Autodesk Inventor part; units mm, degrees
(part 2 of 3)
  line L371 (21.6648, -2.3732) -> (20.3723, -2.3732)
  line L372 (20.3723, -2.3732) -> (20.3723, 1.7763)
  line L373 (20.3723, 1.7763) -> (21.6648, 1.7763)
  line L374 (21.6648, 1.7763) -> (21.6648, -2.3732)
  line L375 (21.7049, 2.3691) -> (20.3366, 2.3691)
  line L376 (20.3366, 2.3691) -> (20.3366, 3.3764)
  line L377 (20.3366, 3.3764) -> (21.7049, 3.3764)
  line L378 (21.7049, 3.3764) -> (21.7049, 2.3691)
  spline S238 degree 2 poles (24.9408, -1.932) (24.8071, -2.0434) (24.5976, -2.2217) (24.4193, -2.3108) knots 0 0 0 1 2 2 2
  spline S239 degree 2 poles (24.4193, -2.3108) (24.2455, -2.3955) (23.9156, -2.4847) (23.6215, -2.4847) knots 0 0 0 1 2 2 2
  spline S240 degree 2 poles (23.6215, -2.4847) (23.0688, -2.4847) (22.3423, -1.7448) (22.3423, -1.1832) knots 0 0 0 1 2 2 2
  spline S241 degree 2 poles (22.3423, -1.1832) (22.3423, -0.7241) (22.7122, -0.1536) (23.0599, 0.0113) knots 0 0 0 1 2 2 2
  spline S242 degree 2 poles (23.0599, 0.0113) (23.412, 0.1807) (24.3881, 0.3144) (24.9497, 0.35) knots 0 0 0 1 2 2 2
  line L379 (24.9497, 0.35) -> (24.9497, 0.3723)
  spline S243 degree 2 poles (24.9497, 0.3723) (24.9497, 0.7155) (24.4416, 0.9785) (23.9335, 0.9785) knots 0 0 0 1 2 2 2
  spline S244 degree 2 poles (23.9335, 0.9785) (23.7062, 0.9785) (23.0911, 0.8136) (22.8014, 0.6843) knots 0 0 0 1 2 2 2
  line L380 (22.8014, 0.6843) -> (22.69, 0.6843)
  line L381 (22.69, 0.6843) -> (22.69, 1.6871)
  spline S245 degree 2 poles (22.69, 1.6871) (22.8816, 1.7406) (23.7374, 1.8922) (24.1741, 1.8922) knots 0 0 0 1 2 2 2
  spline S246 degree 2 poles (24.1741, 1.8922) (25.2438, 1.8922) (26.2244, 1.179) (26.2244, 0.4481) knots 0 0 0 1 2 2 2
  line L382 (26.2244, 0.4481) -> (26.2244, -2.3732)
  line L383 (26.2244, -2.3732) -> (24.9408, -2.3732)
  line L384 (24.9408, -2.3732) -> (24.9408, -1.932)
  line L385 (24.9408, -1.2902) -> (24.9408, -0.43)
  spline S247 degree 2 poles (24.9408, -0.43) (24.6109, -0.4612) (24.2053, -0.5102) (24.0092, -0.5815) knots 0 0 0 1 2 2 2
  spline S248 degree 2 poles (24.0092, -0.5815) (23.8354, -0.6394) (23.6482, -0.8801) (23.6482, -1.0762) knots 0 0 0 1 2 2 2
  spline S249 degree 2 poles (23.6482, -1.0762) (23.6482, -1.3659) (23.9647, -1.5843) (24.2722, -1.5843) knots 0 0 0 1 2 2 2
  spline S250 degree 2 poles (24.2722, -1.5843) (24.4416, -1.5843) (24.7981, -1.4283) (24.9408, -1.2902) knots 0 0 0 1 2 2 2
  line L386 (31.3366, -2.3732) -> (29.7989, -2.3732)
  line L387 (29.7989, -2.3732) -> (28.6758, -0.5726)
  line L388 (28.6758, -0.5726) -> (28.4752, -0.84)
  line L389 (28.4752, -0.84) -> (28.4752, -2.3732)
  line L390 (28.4752, -2.3732) -> (27.1827, -2.3732)
  line L391 (27.1827, -2.3732) -> (27.1827, 3.3719)
  line L392 (27.1827, 3.3719) -> (28.4752, 3.3719)
  line L393 (28.4752, 3.3719) -> (28.4752, 0.1539)
  line L394 (28.4752, 0.1539) -> (29.7009, 1.7763)
  line L395 (29.7009, 1.7763) -> (31.2297, 1.7763)
  line L396 (31.2297, 1.7763) -> (29.7767, -0.011)
  line L397 (29.7767, -0.011) -> (31.3366, -2.3732)
  spline S251 degree 2 poles (-44.3619, -7.6626) (-44.3619, -8.0459) (-44.6071, -8.7412) (-44.8344, -8.973) knots 0 0 0 1 2 2 2
  spline S252 degree 2 poles (-44.8344, -8.973) (-44.9725, -9.1201) (-45.3113, -9.3608) (-45.5118, -9.4454) knots 0 0 0 1 2 2 2
  spline S253 degree 2 poles (-45.5118, -9.4454) (-45.7169, -9.5301) (-46.1938, -9.6282) (-46.4879, -9.6282) knots 0 0 0 1 2 2 2
  line L398 (-46.4879, -9.6282) -> (-47.21, -9.6282)
  line L399 (-47.21, -9.6282) -> (-47.21, -11.4288)
  line L400 (-47.21, -11.4288) -> (-48.5917, -11.4288)
  line L401 (-48.5917, -11.4288) -> (-48.5917, -5.9288)
  line L402 (-48.5917, -5.9288) -> (-46.4567, -5.9288)
  spline S254 degree 2 poles (-46.4567, -5.9288) (-45.9843, -5.9288) (-45.2934, -6.1027) (-45.0126, -6.2899) knots 0 0 0 1 2 2 2
  spline S255 degree 2 poles (-45.0126, -6.2899) (-44.7007, -6.4993) (-44.3619, -7.1857) (-44.3619, -7.6626) knots 0 0 0 1 2 2 2
  spline S256 degree 2 poles (-45.7793, -7.6983) (-45.7793, -7.4621) (-46.0021, -7.1278) (-46.1536, -7.0654) knots 0 0 0 1 2 2 2
  spline S257 degree 2 poles (-46.1536, -7.0654) (-46.3498, -6.9807) (-46.7063, -6.954) (-47.0139, -6.954) knots 0 0 0 1 2 2 2
  line L403 (-47.0139, -6.954) -> (-47.21, -6.954)
  line L404 (-47.21, -6.954) -> (-47.21, -8.6031)
  line L405 (-47.21, -8.6031) -> (-47.1119, -8.6031)
  spline S258 degree 2 poles (-47.1119, -8.6031) (-46.9203, -8.6031) (-46.5726, -8.5941) (-46.4434, -8.5719) knots 0 0 0 1 2 2 2
  spline S259 degree 2 poles (-46.4434, -8.5719) (-46.3319, -8.554) (-46.0868, -8.4471) (-46.0199, -8.3802) knots 0 0 0 1 2 2 2
  spline S260 degree 2 poles (-46.0199, -8.3802) (-45.8773, -8.2465) (-45.7793, -7.9479) (-45.7793, -7.6983) knots 0 0 0 1 2 2 2
  spline S261 degree 2 poles (-39.7177, -9.3563) (-39.7177, -10.3814) (-40.8364, -11.5581) (-41.8571, -11.5581) knots 0 0 0 1 2 2 2
  spline S262 degree 2 poles (-41.8571, -11.5581) (-42.8733, -11.5581) (-44.0009, -10.3814) (-44.0009, -9.3563) knots 0 0 0 1 2 2 2
  spline S263 degree 2 poles (-44.0009, -9.3563) (-44.0009, -8.3223) (-42.8733, -7.1501) (-41.8571, -7.1501) knots 0 0 0 1 2 2 2
  spline S264 degree 2 poles (-41.8571, -7.1501) (-40.8408, -7.1501) (-39.7177, -8.3267) (-39.7177, -9.3563) knots 0 0 0 1 2 2 2
  spline S265 degree 2 poles (-41.0414, -9.3652) (-41.0414, -8.9953) (-41.1618, -8.5006) (-41.2687, -8.3535) knots 0 0 0 1 2 2 2
  spline S266 degree 2 poles (-41.2687, -8.3535) (-41.3846, -8.1975) (-41.6743, -8.0771) (-41.8571, -8.0771) knots 0 0 0 1 2 2 2
  spline S267 degree 2 poles (-41.8571, -8.0771) (-42.0353, -8.0771) (-42.3161, -8.1841) (-42.432, -8.3356) knots 0 0 0 1 2 2 2
  spline S268 degree 2 poles (-42.432, -8.3356) (-42.5434, -8.4783) (-42.6771, -8.9819) (-42.6771, -9.3652) knots 0 0 0 1 2 2 2
  spline S269 degree 2 poles (-42.6771, -9.3652) (-42.6771, -9.7441) (-42.5524, -10.2121) (-42.4498, -10.3547) knots 0 0 0 1 2 2 2
  spline S270 degree 2 poles (-42.4498, -10.3547) (-42.3473, -10.4973) (-42.0353, -10.631) (-41.8481, -10.631) knots 0 0 0 1 2 2 2
  spline S271 degree 2 poles (-41.8481, -10.631) (-41.6921, -10.631) (-41.3712, -10.4973) (-41.2732, -10.3636) knots 0 0 0 1 2 2 2
  spline S272 degree 2 poles (-41.2732, -10.3636) (-41.1618, -10.2076) (-41.0414, -9.7574) (-41.0414, -9.3652) knots 0 0 0 1 2 2 2
  line L406 (-35.2606, -11.4288) -> (-36.5532, -11.4288)
  line L407 (-36.5532, -11.4288) -> (-36.5532, -10.9965)
  spline S273 degree 2 poles (-36.5532, -10.9965) (-36.678, -11.099) (-36.9989, -11.3352) (-37.1237, -11.3976) knots 0 0 0 1 2 2 2
  spline S274 degree 2 poles (-37.1237, -11.3976) (-37.2752, -11.4689) (-37.5783, -11.5447) (-37.7878, -11.5447) knots 0 0 0 1 2 2 2
  spline S275 degree 2 poles (-37.7878, -11.5447) (-38.4964, -11.5447) (-39.3254, -10.3681) (-39.3254, -9.3875) knots 0 0 0 1 2 2 2
  spline S276 degree 2 poles (-39.3254, -9.3875) (-39.3254, -8.8437) (-39.0447, -8.0459) (-38.7995, -7.7518) knots 0 0 0 1 2 2 2
  spline S277 degree 2 poles (-38.7995, -7.7518) (-38.5722, -7.4799) (-37.9304, -7.1679) (-37.5738, -7.1679) knots 0 0 0 1 2 2 2
  spline S278 degree 2 poles (-37.5738, -7.1679) (-37.2485, -7.1679) (-36.8295, -7.3061) (-36.5532, -7.4487) knots 0 0 0 1 2 2 2
  line L408 (-36.5532, -7.4487) -> (-36.5532, -5.6837)
  line L409 (-36.5532, -5.6837) -> (-35.2606, -5.6837)
  line L410 (-35.2606, -5.6837) -> (-35.2606, -11.4288)
  line L411 (-36.5532, -10.2878) -> (-36.5532, -8.251)
  spline S279 degree 2 poles (-36.5532, -8.251) (-36.6468, -8.2019) (-36.9588, -8.1395) (-37.0702, -8.1395) knots 0 0 0 1 2 2 2
  spline S280 degree 2 poles (-37.0702, -8.1395) (-37.5337, -8.1395) (-38.0017, -8.7903) (-38.0017, -9.3741) knots 0 0 0 1 2 2 2
  spline S281 degree 2 poles (-38.0017, -9.3741) (-38.0017, -9.9892) (-37.6273, -10.5374) (-37.2128, -10.5374) knots 0 0 0 1 2 2 2
  spline S282 degree 2 poles (-37.2128, -10.5374) (-37.0434, -10.5374) (-36.6958, -10.4037) (-36.5532, -10.2878) knots 0 0 0 1 2 2 2
  spline S283 degree 2 poles (-28.0759, -9.3563) (-28.0759, -10.3814) (-29.1946, -11.5581) (-30.2152, -11.5581) knots 0 0 0 1 2 2 2
  spline S284 degree 2 poles (-30.2152, -11.5581) (-31.2314, -11.5581) (-32.3591, -10.3814) (-32.3591, -9.3563) knots 0 0 0 1 2 2 2
  spline S285 degree 2 poles (-32.3591, -9.3563) (-32.3591, -8.3223) (-31.2314, -7.1501) (-30.2152, -7.1501) knots 0 0 0 1 2 2 2
  spline S286 degree 2 poles (-30.2152, -7.1501) (-29.199, -7.1501) (-28.0759, -8.3267) (-28.0759, -9.3563) knots 0 0 0 1 2 2 2
  spline S287 degree 2 poles (-29.3996, -9.3652) (-29.3996, -8.9953) (-29.5199, -8.5006) (-29.6269, -8.3535) knots 0 0 0 1 2 2 2
  spline S288 degree 2 poles (-29.6269, -8.3535) (-29.7428, -8.1975) (-30.0325, -8.0771) (-30.2152, -8.0771) knots 0 0 0 1 2 2 2
  spline S289 degree 2 poles (-30.2152, -8.0771) (-30.3935, -8.0771) (-30.6743, -8.1841) (-30.7902, -8.3356) knots 0 0 0 1 2 2 2
  spline S290 degree 2 poles (-30.7902, -8.3356) (-30.9016, -8.4783) (-31.0353, -8.9819) (-31.0353, -9.3652) knots 0 0 0 1 2 2 2
  spline S291 degree 2 poles (-31.0353, -9.3652) (-31.0353, -9.7441) (-30.9105, -10.2121) (-30.808, -10.3547) knots 0 0 0 1 2 2 2
  spline S292 degree 2 poles (-30.808, -10.3547) (-30.7055, -10.4973) (-30.3935, -10.631) (-30.2063, -10.631) knots 0 0 0 1 2 2 2
  spline S293 degree 2 poles (-30.2063, -10.631) (-30.0503, -10.631) (-29.7294, -10.4973) (-29.6314, -10.3636) knots 0 0 0 1 2 2 2
  spline S294 degree 2 poles (-29.6314, -10.3636) (-29.5199, -10.2076) (-29.3996, -9.7574) (-29.3996, -9.3652) knots 0 0 0 1 2 2 2
  spline S295 degree 2 poles (-23.3246, -9.2984) (-23.3246, -10.2923) (-24.3319, -11.5091) (-25.0718, -11.5091) knots 0 0 0 1 2 2 2
  spline S296 degree 2 poles (-25.0718, -11.5091) (-25.3793, -11.5091) (-25.8384, -11.3709) (-26.0969, -11.2194) knots 0 0 0 1 2 2 2
  line L412 (-26.0969, -11.2194) -> (-26.0969, -12.9487)
  line L413 (-26.0969, -12.9487) -> (-27.3895, -12.9487)
  line L414 (-27.3895, -12.9487) -> (-27.3895, -7.2793)
  line L415 (-27.3895, -7.2793) -> (-26.0969, -7.2793)
  line L416 (-26.0969, -7.2793) -> (-26.0969, -7.7161)
  spline S297 degree 2 poles (-26.0969, -7.7161) (-25.8117, -7.471) (-25.2233, -7.1679) (-24.8356, -7.1679) knots 0 0 0 1 2 2 2
  spline S298 degree 2 poles (-24.8356, -7.1679) (-24.1135, -7.1679) (-23.3246, -8.3134) (-23.3246, -9.2984) knots 0 0 0 1 2 2 2
  spline S299 degree 2 poles (-24.6484, -9.3251) (-24.6484, -8.7189) (-25.0228, -8.1752) (-25.415, -8.1752) knots 0 0 0 1 2 2 2
  spline S300 degree 2 poles (-25.415, -8.1752) (-25.5888, -8.1752) (-25.932, -8.2866) (-26.0969, -8.398) knots 0 0 0 1 2 2 2
  line L417 (-26.0969, -8.398) -> (-26.0969, -10.4795)
  spline S301 degree 2 poles (-26.0969, -10.4795) (-25.9944, -10.5241) (-25.7448, -10.5597) (-25.5754, -10.5597) knots 0 0 0 1 2 2 2
  spline S302 degree 2 poles (-25.5754, -10.5597) (-25.1075, -10.5597) (-24.6484, -9.9446) (-24.6484, -9.3251) knots 0 0 0 1 2 2 2
  line L418 (-21.3368, -11.4288) -> (-22.6293, -11.4288)
  line L419 (-22.6293, -11.4288) -> (-22.6293, -7.2793)
  line L420 (-22.6293, -7.2793) -> (-21.3368, -7.2793)
  line L421 (-21.3368, -7.2793) -> (-21.3368, -11.4288)
  line L422 (-21.2967, -6.6865) -> (-22.665, -6.6865)
  line L423 (-22.665, -6.6865) -> (-22.665, -5.6792)
  line L424 (-22.665, -5.6792) -> (-21.2967, -5.6792)
  line L425 (-21.2967, -5.6792) -> (-21.2967, -6.6865)
  spline S303 degree 2 poles (-18.2213, -11.5403) (-19.398, -11.5403) (-20.6504, -10.4171) (-20.6504, -9.3786) knots 0 0 0 1 2 2 2
  spline S304 degree 2 poles (-20.6504, -9.3786) (-20.6504, -8.3624) (-19.4827, -7.1501) (-18.4308, -7.1501) knots 0 0 0 1 2 2 2
  spline S305 degree 2 poles (-18.4308, -7.1501) (-17.4814, -7.1501) (-16.5187, -8.1796) (-16.5187, -9.1335) knots 0 0 0 1 2 2 2
  line L426 (-16.5187, -9.1335) -> (-16.5187, -9.6014)
  line L427 (-16.5187, -9.6014) -> (-19.3579, -9.6014)
  spline S306 degree 2 poles (-19.3579, -9.6014) (-19.34, -9.8911) (-19.1306, -10.2745) (-18.9612, -10.3903) knots 0 0 0 1 2 2 2
  spline S307 degree 2 poles (-18.9612, -10.3903) (-18.7963, -10.5062) (-18.3506, -10.6043) (-18.0876, -10.6043) knots 0 0 0 1 2 2 2
  spline S308 degree 2 poles (-18.0876, -10.6043) (-17.8648, -10.6043) (-17.428, -10.5062) (-17.2452, -10.4215) knots 0 0 0 1 2 2 2
  spline S309 degree 2 poles (-17.2452, -10.4215) (-17.0848, -10.3547) (-16.8173, -10.1898) (-16.7327, -10.1274) knots 0 0 0 1 2 2 2
  line L428 (-16.7327, -10.1274) -> (-16.5945, -10.1274)
  line L429 (-16.5945, -10.1274) -> (-16.5945, -11.1971)
  spline S310 degree 2 poles (-16.5945, -11.1971) (-16.7549, -11.2595) (-17.0135, -11.3664) (-17.2452, -11.4199) knots 0 0 0 1 2 2 2
  spline S311 degree 2 poles (-17.2452, -11.4199) (-17.4547, -11.4779) (-17.9004, -11.5403) (-18.2213, -11.5403) knots 0 0 0 1 2 2 2
  spline S312 degree 2 poles (-17.7934, -8.8215) (-17.8024, -8.4114) (-18.1634, -7.9791) (-18.5333, -7.9791) knots 0 0 0 1 2 2 2
  spline S313 degree 2 poles (-18.5333, -7.9791) (-18.9122, -7.9791) (-19.34, -8.4337) (-19.3623, -8.8215) knots 0 0 0 1 2 2 2
  line L430 (-19.3623, -8.8215) -> (-17.7934, -8.8215)
  line L431 (-11.7006, -11.4288) -> (-13.2383, -11.4288)
  line L432 (-13.2383, -11.4288) -> (-14.3615, -9.6282)
  line L433 (-14.3615, -9.6282) -> (-14.5621, -9.8956)
  line L434 (-14.5621, -9.8956) -> (-14.5621, -11.4288)
  line L435 (-14.5621, -11.4288) -> (-15.8546, -11.4288)
  line L436 (-15.8546, -11.4288) -> (-15.8546, -5.6837)
  line L437 (-15.8546, -5.6837) -> (-14.5621, -5.6837)
  line L438 (-14.5621, -5.6837) -> (-14.5621, -8.9017)
  line L439 (-14.5621, -8.9017) -> (-13.3364, -7.2793)
  line L440 (-13.3364, -7.2793) -> (-11.8076, -7.2793)
  line L441 (-11.8076, -7.2793) -> (-13.2606, -9.0666)
  line L442 (-13.2606, -9.0666) -> (-11.7006, -11.4288)
  spline S314 degree 2 poles (-9.0086, -10.9876) (-9.1423, -11.099) (-9.3518, -11.2773) (-9.5301, -11.3664) knots 0 0 0 1 2 2 2
  spline S315 degree 2 poles (-9.5301, -11.3664) (-9.7039, -11.4511) (-10.0337, -11.5403) (-10.3279, -11.5403) knots 0 0 0 1 2 2 2
  spline S316 degree 2 poles (-10.3279, -11.5403) (-10.8806, -11.5403) (-11.6071, -10.8004) (-11.6071, -10.2388) knots 0 0 0 1 2 2 2
  spline S317 degree 2 poles (-11.6071, -10.2388) (-11.6071, -9.7797) (-11.2371, -9.2092) (-10.8895, -9.0443) knots 0 0 0 1 2 2 2
  spline S318 degree 2 poles (-10.8895, -9.0443) (-10.5374, -8.8749) (-9.5613, -8.7412) (-8.9997, -8.7056) knots 0 0 0 1 2 2 2
  line L443 (-8.9997, -8.7056) -> (-8.9997, -8.6833)
  spline S319 degree 2 poles (-8.9997, -8.6833) (-8.9997, -8.3401) (-9.5078, -8.0771) (-10.0159, -8.0771) knots 0 0 0 1 2 2 2
  spline S320 degree 2 poles (-10.0159, -8.0771) (-10.2432, -8.0771) (-10.8583, -8.242) (-11.148, -8.3713) knots 0 0 0 1 2 2 2
  line L444 (-11.148, -8.3713) -> (-11.2594, -8.3713)
  line L445 (-11.2594, -8.3713) -> (-11.2594, -7.3685)
  spline S321 degree 2 poles (-11.2594, -7.3685) (-11.0677, -7.315) (-10.212, -7.1634) (-9.7752, -7.1634) knots 0 0 0 1 2 2 2
  spline S322 degree 2 poles (-9.7752, -7.1634) (-8.7055, -7.1634) (-7.725, -7.8766) (-7.725, -8.6075) knots 0 0 0 1 2 2 2
  line L446 (-7.725, -8.6075) -> (-7.725, -11.4288)
  line L447 (-7.725, -11.4288) -> (-9.0086, -11.4288)
  line L448 (-9.0086, -11.4288) -> (-9.0086, -10.9876)
  spline S323 degree 2 poles (-7.9746, -11.4288) (-8.1127, -11.5358) (-8.2464, -11.7676) (-8.2464, -11.8745) knots 0 0 0 1 2 2 2
  spline S324 degree 2 poles (-8.2464, -11.8745) (-8.2464, -11.9191) (-8.2197, -11.9993) (-8.1885, -12.035) knots 0 0 0 1 2 2 2
  spline S325 degree 2 poles (-8.1885, -12.035) (-8.1484, -12.0751) (-8.0637, -12.1152) (-7.9835, -12.1152) knots 0 0 0 1 2 2 2
  spline S326 degree 2 poles (-7.9835, -12.1152) (-7.93, -12.1152) (-7.8007, -12.084) (-7.7562, -12.0706) knots 0 0 0 1 2 2 2
  line L449 (-7.7562, -12.0706) -> (-7.7205, -12.0706)
  line L450 (-7.7205, -12.0706) -> (-7.7205, -12.8373)
  spline S327 degree 2 poles (-7.7205, -12.8373) (-7.872, -12.8952) (-8.2687, -12.9487) (-8.3846, -12.9487) knots 0 0 0 1 2 2 2
  spline S328 degree 2 poles (-8.3846, -12.9487) (-8.7323, -12.9487) (-9.1646, -12.5832) (-9.1646, -12.3113) knots 0 0 0 1 2 2 2
  spline S329 degree 2 poles (-9.1646, -12.3113) (-9.1646, -12.0305) (-8.8972, -11.567) (-8.7367, -11.4288) knots 0 0 0 1 2 2 2
  line L451 (-8.7367, -11.4288) -> (-7.9746, -11.4288)
  line L452 (-9.0086, -10.3458) -> (-9.0086, -9.4856)
  spline S330 degree 2 poles (-9.0086, -9.4856) (-9.3384, -9.5168) (-9.744, -9.5658) (-9.9401, -9.6371) knots 0 0 0 1 2 2 2
  spline S331 degree 2 poles (-9.9401, -9.6371) (-10.1139, -9.695) (-10.3011, -9.9357) (-10.3011, -10.1318) knots 0 0 0 1 2 2 2
  spline S332 degree 2 poles (-10.3011, -10.1318) (-10.3011, -10.4215) (-9.9847, -10.6399) (-9.6771, -10.6399) knots 0 0 0 1 2 2 2
  spline S333 degree 2 poles (-9.6771, -10.6399) (-9.5078, -10.6399) (-9.1512, -10.4839) (-9.0086, -10.3458) knots 0 0 0 1 2 2 2
  line L453 (0.4002, -11.4288) -> (0.4002, -9.3563)
  spline S334 degree 2 poles (0.4002, -9.3563) (0.4002, -9.0488) (0.378, -8.6298) (0.3245, -8.4961) knots 0 0 0 1 2 2 2
  spline S335 degree 2 poles (0.3245, -8.4961) (0.2665, -8.3624) (0.0348, -8.242) (-0.1747, -8.242) knots 0 0 0 1 2 2 2
  spline S336 degree 2 poles (-0.1747, -8.242) (-0.3218, -8.242) (-0.6071, -8.3713) (-0.7764, -8.4916) knots 0 0 0 1 2 2 2
  line L454 (-0.7764, -8.4916) -> (-0.7764, -11.4288)
  line L455 (-0.7764, -11.4288) -> (-2.0779, -11.4288)
  line L456 (-2.0779, -11.4288) -> (-2.0779, -9.3563)
  spline S337 degree 2 poles (-2.0779, -9.3563) (-2.0779, -9.0532) (-2.1046, -8.6298) (-2.1581, -8.4961) knots 0 0 0 1 2 2 2
  spline S338 degree 2 poles (-2.1581, -8.4961) (-2.216, -8.3624) (-2.4478, -8.242) (-2.6573, -8.242) knots 0 0 0 1 2 2 2
  spline S339 degree 2 poles (-2.6573, -8.242) (-2.8133, -8.242) (-3.1208, -8.3891) (-3.2635, -8.4916) knots 0 0 0 1 2 2 2
  line L457 (-3.2635, -8.4916) -> (-3.2635, -11.4288)
  line L458 (-3.2635, -11.4288) -> (-4.556, -11.4288)
  line L459 (-4.556, -11.4288) -> (-4.556, -7.2793)
  line L460 (-4.556, -7.2793) -> (-3.2635, -7.2793)
  line L461 (-3.2635, -7.2793) -> (-3.2635, -7.7384)
  spline S340 degree 2 poles (-3.2635, -7.7384) (-2.947, -7.471) (-2.381, -7.1679) (-2.0289, -7.1679) knots 0 0 0 1 2 2 2
  spline S341 degree 2 poles (-2.0289, -7.1679) (-1.65, -7.1679) (-1.0706, -7.5289) (-0.919, -7.8899) knots 0 0 0 1 2 2 2
  spline S342 degree 2 poles (-0.919, -7.8899) (-0.5491, -7.5423) (0.1105, -7.1679) (0.4493, -7.1679) knots 0 0 0 1 2 2 2
  spline S343 degree 2 poles (0.4493, -7.1679) (0.739, -7.1679) (1.1981, -7.3506) (1.3541, -7.5378) knots 0 0 0 1 2 2 2
  spline S344 degree 2 poles (1.3541, -7.5378) (1.5279, -7.7384) (1.7017, -8.2866) (1.7017, -8.7279) knots 0 0 0 1 2 2 2
  line L462 (1.7017, -8.7279) -> (1.7017, -11.4288)
  line L463 (1.7017, -11.4288) -> (0.4002, -11.4288)
  spline S345 degree 2 poles (4.786, -11.5403) (3.6093, -11.5403) (2.3569, -10.4171) (2.3569, -9.3786) knots 0 0 0 1 2 2 2
  spline S346 degree 2 poles (2.3569, -9.3786) (2.3569, -8.3624) (3.5246, -7.1501) (4.5765, -7.1501) knots 0 0 0 1 2 2 2
  spline S347 degree 2 poles (4.5765, -7.1501) (5.5259, -7.1501) (6.4886, -8.1796) (6.4886, -9.1335) knots 0 0 0 1 2 2 2
  line L464 (6.4886, -9.1335) -> (6.4886, -9.6014)
  line L465 (6.4886, -9.6014) -> (3.6494, -9.6014)
  spline S348 degree 2 poles (3.6494, -9.6014) (3.6673, -9.8911) (3.8767, -10.2745) (4.0461, -10.3903) knots 0 0 0 1 2 2 2
  spline S349 degree 2 poles (4.0461, -10.3903) (4.211, -10.5062) (4.6567, -10.6043) (4.9197, -10.6043) knots 0 0 0 1 2 2 2
  spline S350 degree 2 poles (4.9197, -10.6043) (5.1425, -10.6043) (5.5793, -10.5062) (5.7621, -10.4215) knots 0 0 0 1 2 2 2
  spline S351 degree 2 poles (5.7621, -10.4215) (5.9225, -10.3547) (6.19, -10.1898) (6.2746, -10.1274) knots 0 0 0 1 2 2 2
  line L466 (6.2746, -10.1274) -> (6.4128, -10.1274)
  line L467 (6.4128, -10.1274) -> (6.4128, -11.1971)
  spline S352 degree 2 poles (6.4128, -11.1971) (6.2523, -11.2595) (5.9938, -11.3664) (5.7621, -11.4199) knots 0 0 0 1 2 2 2
  spline S353 degree 2 poles (5.7621, -11.4199) (5.5526, -11.4779) (5.1069, -11.5403) (4.786, -11.5403) knots 0 0 0 1 2 2 2
  spline S354 degree 2 poles (5.2139, -8.8215) (5.2049, -8.4114) (4.8439, -7.9791) (4.474, -7.9791) knots 0 0 0 1 2 2 2
  spline S355 degree 2 poles (4.474, -7.9791) (4.0951, -7.9791) (3.6673, -8.4337) (3.645, -8.8215) knots 0 0 0 1 2 2 2
  line L468 (3.645, -8.8215) -> (5.2139, -8.8215)
  line L469 (9.9383, -8.505) -> (9.8314, -8.505)
  spline S356 degree 2 poles (9.8314, -8.505) (9.7556, -8.4783) (9.4748, -8.4515) (9.3054, -8.4515) knots 0 0 0 1 2 2 2
  spline S357 degree 2 poles (9.3054, -8.4515) (9.1049, -8.4515) (8.6547, -8.5719) (8.4452, -8.6521) knots 0 0 0 1 2 2 2
  line L470 (8.4452, -8.6521) -> (8.4452, -11.4288)
  line L471 (8.4452, -11.4288) -> (7.1527, -11.4288)
  line L472 (7.1527, -11.4288) -> (7.1527, -7.2793)
  line L473 (7.1527, -7.2793) -> (8.4452, -7.2793)
  line L474 (8.4452, -7.2793) -> (8.4452, -7.8766)
  spline S358 degree 2 poles (8.4452, -7.8766) (8.5344, -7.7963) (8.8464, -7.5467) (8.9756, -7.471) knots 0 0 0 1 2 2 2
  spline S359 degree 2 poles (8.9756, -7.471) (9.1182, -7.3863) (9.4926, -7.2659) (9.6575, -7.2659) knots 0 0 0 1 2 2 2
  spline S360 degree 2 poles (9.6575, -7.2659) (9.7199, -7.2659) (9.8759, -7.2749) (9.9383, -7.2793) knots 0 0 0 1 2 2 2
  line L475 (9.9383, -7.2793) -> (9.9383, -8.505)
  line L476 (14.3018, -7.2793) -> (12.2114, -12.9487)
  line L477 (12.2114, -12.9487) -> (10.8208, -12.9487)
  line L478 (10.8208, -12.9487) -> (11.4493, -11.3263)
  line L479 (11.4493, -11.3263) -> (9.9294, -7.2793)
  line L480 (9.9294, -7.2793) -> (11.2844, -7.2793)
  line L481 (11.2844, -7.2793) -> (12.1579, -9.8822)
  line L482 (12.1579, -9.8822) -> (12.9736, -7.2793)
  line L483 (12.9736, -7.2793) -> (14.3018, -7.2793)
  spline S361 degree 2 poles (16.3743, -11.5091) (15.5854, -11.5091) (14.8634, -10.8583) (14.8634, -10.1185) knots 0 0 0 1 2 2 2
  line L484 (14.8634, -10.1185) -> (14.8634, -8.1796)
  line L485 (14.8634, -8.1796) -> (14.3686, -8.1796)
  line L486 (14.3686, -8.1796) -> (14.3686, -7.2793)
  line L487 (14.3686, -7.2793) -> (14.8634, -7.2793)
  line L488 (14.8634, -7.2793) -> (14.8634, -6.0937)
  line L489 (14.8634, -6.0937) -> (16.1559, -6.0937)
  line L490 (16.1559, -6.0937) -> (16.1559, -7.2793)
  line L491 (16.1559, -7.2793) -> (17.4039, -7.2793)
  line L492 (17.4039, -7.2793) -> (17.4039, -8.1796)
  line L493 (17.4039, -8.1796) -> (16.1559, -8.1796)
  line L494 (16.1559, -8.1796) -> (16.1559, -9.6549)
  spline S362 degree 2 poles (16.1559, -9.6549) (16.1559, -9.8733) (16.1648, -10.1987) (16.2183, -10.3279) knots 0 0 0 1 2 2 2
  spline S363 degree 2 poles (16.2183, -10.3279) (16.2718, -10.4572) (16.5348, -10.6087) (16.7844, -10.6087) knots 0 0 0 1 2 2 2
  spline S364 degree 2 poles (16.7844, -10.6087) (16.8913, -10.6087) (17.2256, -10.5196) (17.2925, -10.4839) knots 0 0 0 1 2 2 2
  line L495 (17.2925, -10.4839) -> (17.4039, -10.4839)
  line L496 (17.4039, -10.4839) -> (17.4039, -11.3932)
  spline S365 degree 2 poles (17.4039, -11.3932) (17.1944, -11.4467) (16.722, -11.5091) (16.3743, -11.5091) knots 0 0 0 1 2 2 2
  spline S366 degree 2 poles (21.91, -9.3563) (21.91, -10.3814) (20.7912, -11.5581) (19.7706, -11.5581) knots 0 0 0 1 2 2 2
  spline S367 degree 2 poles (19.7706, -11.5581) (18.7544, -11.5581) (17.6267, -10.3814) (17.6267, -9.3563) knots 0 0 0 1 2 2 2
  spline S368 degree 2 poles (17.6267, -9.3563) (17.6267, -8.3223) (18.7544, -7.1501) (19.7706, -7.1501) knots 0 0 0 1 2 2 2
  spline S369 degree 2 poles (19.7706, -7.1501) (20.7868, -7.1501) (21.91, -8.3267) (21.91, -9.3563) knots 0 0 0 1 2 2 2
  spline S370 degree 2 poles (20.5862, -9.3652) (20.5862, -8.9953) (20.4659, -8.5006) (20.3589, -8.3535) knots 0 0 0 1 2 2 2
  spline S371 degree 2 poles (20.3589, -8.3535) (20.243, -8.1975) (19.9533, -8.0771) (19.7706, -8.0771) knots 0 0 0 1 2 2 2
  spline S372 degree 2 poles (19.7706, -8.0771) (19.5923, -8.0771) (19.3115, -8.1841) (19.1956, -8.3356) knots 0 0 0 1 2 2 2
  spline S373 degree 2 poles (19.1956, -8.3356) (19.0842, -8.4783) (18.9505, -8.9819) (18.9505, -9.3652) knots 0 0 0 1 2 2 2
  spline S374 degree 2 poles (18.9505, -9.3652) (18.9505, -9.7441) (19.0753, -10.2121) (19.1778, -10.3547) knots 0 0 0 1 2 2 2
  spline S375 degree 2 poles (19.1778, -10.3547) (19.2803, -10.4973) (19.5923, -10.631) (19.7795, -10.631) knots 0 0 0 1 2 2 2
  spline S376 degree 2 poles (19.7795, -10.631) (19.9355, -10.631) (20.2564, -10.4973) (20.3545, -10.3636) knots 0 0 0 1 2 2 2
  spline S377 degree 2 poles (20.3545, -10.3636) (20.4659, -10.2076) (20.5862, -9.7574) (20.5862, -9.3652) knots 0 0 0 1 2 2 2
  line L497 (25.382, -8.505) -> (25.275, -8.505)
  spline S378 degree 2 poles (25.275, -8.505) (25.1993, -8.4783) (24.9185, -8.4515) (24.7491, -8.4515) knots 0 0 0 1 2 2 2
  spline S379 degree 2 poles (24.7491, -8.4515) (24.5485, -8.4515) (24.0984, -8.5719) (23.8889, -8.6521) knots 0 0 0 1 2 2 2
  line L498 (23.8889, -8.6521) -> (23.8889, -11.4288)
  line L499 (23.8889, -11.4288) -> (22.5964, -11.4288)
  line L500 (22.5964, -11.4288) -> (22.5964, -7.2793)
  line L501 (22.5964, -7.2793) -> (23.8889, -7.2793)
  line L502 (23.8889, -7.2793) -> (23.8889, -7.8766)
  spline S380 degree 2 poles (23.8889, -7.8766) (23.978, -7.7963) (24.29, -7.5467) (24.4193, -7.471) knots 0 0 0 1 2 2 2
  spline S381 degree 2 poles (24.4193, -7.471) (24.5619, -7.3863) (24.9363, -7.2659) (25.1012, -7.2659) knots 0 0 0 1 2 2 2
  spline S382 degree 2 poles (25.1012, -7.2659) (25.1636, -7.2659) (25.3196, -7.2749) (25.382, -7.2793) knots 0 0 0 1 2 2 2
  line L503 (25.382, -7.2793) -> (25.382, -8.505)
  line L504 (29.7455, -7.2793) -> (27.6551, -12.9487)
  line L505 (27.6551, -12.9487) -> (26.2645, -12.9487)
  line L506 (26.2645, -12.9487) -> (26.8929, -11.3263)
  line L507 (26.8929, -11.3263) -> (25.3731, -7.2793)
  line L508 (25.3731, -7.2793) -> (26.728, -7.2793)
  line L509 (26.728, -7.2793) -> (27.6016, -9.8822)
  line L510 (27.6016, -9.8822) -> (28.4173, -7.2793)
  line L511 (28.4173, -7.2793) -> (29.7455, -7.2793)
  spline S383 degree 2 poles (32.2637, -11.5403) (31.7511, -11.5403) (30.8998, -11.2817) (30.5834, -11.0143) knots 0 0 0 1 2 2 2
  spline S384 degree 2 poles (30.5834, -11.0143) (30.2759, -10.7424) (29.9282, -9.9268) (29.9282, -9.3741) knots 0 0 0 1 2 2 2
  spline S385 degree 2 poles (29.9282, -9.3741) (29.9282, -8.7769) (30.3026, -7.9434) (30.628, -7.676) knots 0 0 0 1 2 2 2
  spline S386 degree 2 poles (30.628, -7.676) (30.9355, -7.4175) (31.7734, -7.1679) (32.228, -7.1679) knots 0 0 0 1 2 2 2
  spline S387 degree 2 poles (32.228, -7.1679) (32.5712, -7.1679) (33.2576, -7.3283) (33.6053, -7.5022) knots 0 0 0 1 2 2 2
  line L512 (33.6053, -7.5022) -> (33.6053, -8.6075)
  line L513 (33.6053, -8.6075) -> (33.4404, -8.6075)
  spline S388 degree 2 poles (33.4404, -8.6075) (33.3601, -8.5317) (33.1373, -8.3535) (33.0036, -8.2822) knots 0 0 0 1 2 2 2
  spline S389 degree 2 poles (33.0036, -8.2822) (32.8609, -8.2019) (32.5088, -8.095) (32.2904, -8.095) knots 0 0 0 1 2 2 2
  spline S390 degree 2 poles (32.2904, -8.095) (31.7957, -8.095) (31.2519, -8.7858) (31.2519, -9.3741) knots 0 0 0 1 2 2 2
  spline S391 degree 2 poles (31.2519, -9.3741) (31.2519, -9.9981) (31.8314, -10.6132) (32.3127, -10.6132) knots 0 0 0 1 2 2 2
  spline S392 degree 2 poles (32.3127, -10.6132) (32.5579, -10.6132) (32.9233, -10.5018) (33.0571, -10.4215) knots 0 0 0 1 2 2 2
  spline S393 degree 2 poles (33.0571, -10.4215) (33.1863, -10.3458) (33.3735, -10.1764) (33.4404, -10.1095) knots 0 0 0 1 2 2 2
  line L514 (33.4404, -10.1095) -> (33.6053, -10.1095)
  line L515 (33.6053, -10.1095) -> (33.6053, -11.2194)
  spline S394 degree 2 poles (33.6053, -11.2194) (33.4938, -11.2684) (33.2041, -11.3932) (33.0526, -11.4333) knots 0 0 0 1 2 2 2
  spline S395 degree 2 poles (33.0526, -11.4333) (32.8654, -11.4868) (32.5356, -11.5403) (32.2637, -11.5403) knots 0 0 0 1 2 2 2
  line L516 (37.5275, -11.4288) -> (33.9039, -11.4288)
  line L517 (33.9039, -11.4288) -> (33.9039, -10.5775)
  line L518 (33.9039, -10.5775) -> (35.8828, -8.251)
  line L519 (35.8828, -8.251) -> (33.993, -8.251)
  line L520 (33.993, -8.251) -> (33.993, -7.2793)
  line L521 (33.993, -7.2793) -> (37.4874, -7.2793)
  line L522 (37.4874, -7.2793) -> (37.4874, -8.1172)
  line L523 (37.4874, -8.1172) -> (35.504, -10.4394)
  line L524 (35.504, -10.4394) -> (37.5275, -10.4394)
  line L525 (37.5275, -10.4394) -> (37.5275, -11.4288)
  line L526 (42.0781, -11.4288) -> (40.7767, -11.4288)
  line L527 (40.7767, -11.4288) -> (40.7767, -9.3741)
  spline S396 degree 2 poles (40.7767, -9.3741) (40.7767, -9.1201) (40.7365, -8.6209) (40.6831, -8.505) knots 0 0 0 1 2 2 2
  spline S397 degree 2 poles (40.6831, -8.505) (40.6162, -8.3624) (40.3666, -8.242) (40.1527, -8.242) knots 0 0 0 1 2 2 2
  spline S398 degree 2 poles (40.1527, -8.242) (39.9967, -8.242) (39.6713, -8.3624) (39.4886, -8.4916) knots 0 0 0 1 2 2 2
  line L528 (39.4886, -8.4916) -> (39.4886, -11.4288)
  line L529 (39.4886, -11.4288) -> (38.196, -11.4288)
  line L530 (38.196, -11.4288) -> (38.196, -7.2793)
  line L531 (38.196, -7.2793) -> (39.4886, -7.2793)
  line L532 (39.4886, -7.2793) -> (39.4886, -7.7384)
  spline S399 degree 2 poles (39.4886, -7.7384) (39.805, -7.471) (40.4067, -7.1679) (40.7722, -7.1679) knots 0 0 0 1 2 2 2
  spline S400 degree 2 poles (40.7722, -7.1679) (41.4051, -7.1679) (42.0781, -7.9702) (42.0781, -8.7279) knots 0 0 0 1 2 2 2
  line L533 (42.0781, -8.7279) -> (42.0781, -11.4288)
  spline S401 degree 2 poles (45.3229, -10.9876) (45.1891, -11.099) (44.9797, -11.2773) (44.8014, -11.3664) knots 0 0 0 1 2 2 2
  spline S402 degree 2 poles (44.8014, -11.3664) (44.6276, -11.4511) (44.2977, -11.5403) (44.0036, -11.5403) knots 0 0 0 1 2 2 2
  spline S403 degree 2 poles (44.0036, -11.5403) (43.4509, -11.5403) (42.7244, -10.8004) (42.7244, -10.2388) knots 0 0 0 1 2 2 2
  spline S404 degree 2 poles (42.7244, -10.2388) (42.7244, -9.7797) (43.0943, -9.2092) (43.442, -9.0443) knots 0 0 0 1 2 2 2
  spline S405 degree 2 poles (43.442, -9.0443) (43.7941, -8.8749) (44.7702, -8.7412) (45.3318, -8.7056) knots 0 0 0 1 2 2 2
  line L534 (45.3318, -8.7056) -> (45.3318, -8.6833)
  spline S406 degree 2 poles (45.3318, -8.6833) (45.3318, -8.3401) (44.8237, -8.0771) (44.3156, -8.0771) knots 0 0 0 1 2 2 2
  spline S407 degree 2 poles (44.3156, -8.0771) (44.0882, -8.0771) (43.4732, -8.242) (43.1835, -8.3713) knots 0 0 0 1 2 2 2
  line L535 (43.1835, -8.3713) -> (43.072, -8.3713)
  line L536 (43.072, -8.3713) -> (43.072, -7.3685)
  spline S408 degree 2 poles (43.072, -7.3685) (43.2637, -7.315) (44.1194, -7.1634) (44.5562, -7.1634) knots 0 0 0 1 2 2 2
  spline S409 degree 2 poles (44.5562, -7.1634) (45.6259, -7.1634) (46.6065, -7.8766) (46.6065, -8.6075) knots 0 0 0 1 2 2 2
  line L537 (46.6065, -8.6075) -> (46.6065, -11.4288)
  line L538 (46.6065, -11.4288) -> (45.3229, -11.4288)
  line L539 (45.3229, -11.4288) -> (45.3229, -10.9876)
  spline S410 degree 2 poles (46.3569, -11.4288) (46.2187, -11.5358) (46.085, -11.7676) (46.085, -11.8745) knots 0 0 0 1 2 2 2
  spline S411 degree 2 poles (46.085, -11.8745) (46.085, -11.9191) (46.1118, -11.9993) (46.1429, -12.035) knots 0 0 0 1 2 2 2
  spline S412 degree 2 poles (46.1429, -12.035) (46.1831, -12.0751) (46.2677, -12.1152) (46.348, -12.1152) knots 0 0 0 1 2 2 2
  spline S413 degree 2 poles (46.348, -12.1152) (46.4015, -12.1152) (46.5307, -12.084) (46.5753, -12.0706) knots 0 0 0 1 2 2 2
  line L540 (46.5753, -12.0706) -> (46.6109, -12.0706)
  line L541 (46.6109, -12.0706) -> (46.6109, -12.8373)
  spline S414 degree 2 poles (46.6109, -12.8373) (46.4594, -12.8952) (46.0627, -12.9487) (45.9468, -12.9487) knots 0 0 0 1 2 2 2
  spline S415 degree 2 poles (45.9468, -12.9487) (45.5992, -12.9487) (45.1669, -12.5832) (45.1669, -12.3113) knots 0 0 0 1 2 2 2
  spline S416 degree 2 poles (45.1669, -12.3113) (45.1669, -12.0305) (45.4343, -11.567) (45.5947, -11.4288) knots 0 0 0 1 2 2 2
  line L542 (45.5947, -11.4288) -> (46.3569, -11.4288)
  line L543 (45.3229, -10.3458) -> (45.3229, -9.4856)
  spline S417 degree 2 poles (45.3229, -9.4856) (44.993, -9.5168) (44.5874, -9.5658) (44.3913, -9.6371) knots 0 0 0 1 2 2 2
  spline S418 degree 2 poles (44.3913, -9.6371) (44.2175, -9.695) (44.0303, -9.9357) (44.0303, -10.1318) knots 0 0 0 1 2 2 2
  spline S419 degree 2 poles (44.0303, -10.1318) (44.0303, -10.4215) (44.3468, -10.6399) (44.6543, -10.6399) knots 0 0 0 1 2 2 2
  spline S420 degree 2 poles (44.6543, -10.6399) (44.8237, -10.6399) (45.1802, -10.4839) (45.3229, -10.3458) knots 0 0 0 1 2 2 2
  line L544 (49.098, -8.7323) -> (47.7921, -8.7323)
  line L545 (47.7921, -8.7323) -> (47.7921, -7.2793)
  line L546 (47.7921, -7.2793) -> (49.098, -7.2793)
  line L547 (49.098, -7.2793) -> (49.098, -8.7323)
  line L548 (49.098, -11.4288) -> (47.7921, -11.4288)
  line L549 (47.7921, -11.4288) -> (47.7921, -9.9758)
  line L550 (47.7921, -9.9758) -> (49.098, -9.9758)
  line L551 (49.098, -9.9758) -> (49.098, -11.4288)
  line L552 (-53.2604, -20.4844) -> (-54.553, -20.4844)
  line L553 (-54.553, -20.4844) -> (-54.553, -20.0521)
  spline S421 degree 2 poles (-54.553, -20.0521) (-54.6778, -20.1546) (-54.9987, -20.3908) (-55.1235, -20.4532) knots 0 0 0 1 2 2 2
  spline S422 degree 2 poles (-55.1235, -20.4532) (-55.275, -20.5246) (-55.5781, -20.6003) (-55.7876, -20.6003) knots 0 0 0 1 2 2 2
  spline S423 degree 2 poles (-55.7876, -20.6003) (-56.4962, -20.6003) (-57.3252, -19.4237) (-57.3252, -18.4431) knots 0 0 0 1 2 2 2
  spline S424 degree 2 poles (-57.3252, -18.4431) (-57.3252, -17.8993) (-57.0444, -17.1015) (-56.7993, -16.8074) knots 0 0 0 1 2 2 2
  spline S425 degree 2 poles (-56.7993, -16.8074) (-56.572, -16.5355) (-55.9302, -16.2235) (-55.5736, -16.2235) knots 0 0 0 1 2 2 2
  spline S426 degree 2 poles (-55.5736, -16.2235) (-55.2483, -16.2235) (-54.8293, -16.3617) (-54.553, -16.5043) knots 0 0 0 1 2 2 2
  line L554 (-54.553, -16.5043) -> (-54.553, -14.7393)
  line L555 (-54.553, -14.7393) -> (-53.2604, -14.7393)
  line L556 (-53.2604, -14.7393) -> (-53.2604, -20.4844)
  line L557 (-54.553, -19.3434) -> (-54.553, -17.3066)
  spline S427 degree 2 poles (-54.553, -17.3066) (-54.6466, -17.2575) (-54.9585, -17.1951) (-55.07, -17.1951) knots 0 0 0 1 2 2 2
  spline S428 degree 2 poles (-55.07, -17.1951) (-55.5335, -17.1951) (-56.0015, -17.8459) (-56.0015, -18.4297) knots 0 0 0 1 2 2 2
  spline S429 degree 2 poles (-56.0015, -18.4297) (-56.0015, -19.0448) (-55.6271, -19.593) (-55.2126, -19.593) knots 0 0 0 1 2 2 2
  spline S430 degree 2 poles (-55.2126, -19.593) (-55.0432, -19.593) (-54.6956, -19.4593) (-54.553, -19.3434) knots 0 0 0 1 2 2 2
  line L558 (-49.4853, -17.5606) -> (-49.5923, -17.5606)
  spline S431 degree 2 poles (-49.5923, -17.5606) (-49.668, -17.5339) (-49.9488, -17.5071) (-50.1182, -17.5071) knots 0 0 0 1 2 2 2
  spline S432 degree 2 poles (-50.1182, -17.5071) (-50.3188, -17.5071) (-50.7689, -17.6275) (-50.9784, -17.7077) knots 0 0 0 1 2 2 2
  line L559 (-50.9784, -17.7077) -> (-50.9784, -20.4844)
  line L560 (-50.9784, -20.4844) -> (-52.2709, -20.4844)
  line L561 (-52.2709, -20.4844) -> (-52.2709, -16.3349)
  line L562 (-52.2709, -16.3349) -> (-50.9784, -16.3349)
  line L563 (-50.9784, -16.3349) -> (-50.9784, -16.9322)
  spline S433 degree 2 poles (-50.9784, -16.9322) (-50.8893, -16.8519) (-50.5773, -16.6023) (-50.448, -16.5266) knots 0 0 0 1 2 2 2
  spline S434 degree 2 poles (-50.448, -16.5266) (-50.3054, -16.4419) (-49.931, -16.3216) (-49.7661, -16.3216) knots 0 0 0 1 2 2 2
  spline S435 degree 2 poles (-49.7661, -16.3216) (-49.7037, -16.3216) (-49.5477, -16.3305) (-49.4853, -16.3349) knots 0 0 0 1 2 2 2
  line L564 (-49.4853, -16.3349) -> (-49.4853, -17.5606)
  line L565 (-45.4829, -20.4844) -> (-46.7754, -20.4844)
  line L566 (-46.7754, -20.4844) -> (-46.7754, -16.3349)
  line L567 (-46.7754, -16.3349) -> (-45.4829, -16.3349)
  line L568 (-45.4829, -16.3349) -> (-45.4829, -20.4844)
  line L569 (-45.4427, -15.7421) -> (-46.8111, -15.7421)
  line L570 (-46.8111, -15.7421) -> (-46.8111, -14.7348)
  line L571 (-46.8111, -14.7348) -> (-45.4427, -14.7348)
  line L572 (-45.4427, -14.7348) -> (-45.4427, -15.7421)
  line L573 (-40.6113, -20.4844) -> (-41.9128, -20.4844)
  line L574 (-41.9128, -20.4844) -> (-41.9128, -18.4297)
  spline S436 degree 2 poles (-41.9128, -18.4297) (-41.9128, -18.1757) (-41.9529, -17.6765) (-42.0064, -17.5606) knots 0 0 0 1 2 2 2
  spline S437 degree 2 poles (-42.0064, -17.5606) (-42.0732, -17.418) (-42.3228, -17.2976) (-42.5367, -17.2976) knots 0 0 0 1 2 2 2
  spline S438 degree 2 poles (-42.5367, -17.2976) (-42.6927, -17.2976) (-43.0181, -17.418) (-43.2009, -17.5472) knots 0 0 0 1 2 2 2
  line L575 (-43.2009, -17.5472) -> (-43.2009, -20.4844)
  line L576 (-43.2009, -20.4844) -> (-44.4934, -20.4844)
  line L577 (-44.4934, -20.4844) -> (-44.4934, -16.3349)
  line L578 (-44.4934, -16.3349) -> (-43.2009, -16.3349)
  line L579 (-43.2009, -16.3349) -> (-43.2009, -16.794)
  spline S439 degree 2 poles (-43.2009, -16.794) (-42.8844, -16.5266) (-42.2827, -16.2235) (-41.9172, -16.2235) knots 0 0 0 1 2 2 2
  spline S440 degree 2 poles (-41.9172, -16.2235) (-41.2843, -16.2235) (-40.6113, -17.0258) (-40.6113, -17.7835) knots 0 0 0 1 2 2 2
  line L580 (-40.6113, -17.7835) -> (-40.6113, -20.4844)
  line L581 (-36.3459, -20.4844) -> (-39.9695, -20.4844)
  line L582 (-39.9695, -20.4844) -> (-39.9695, -19.6331)
  line L583 (-39.9695, -19.6331) -> (-37.9906, -17.3066)
  line L584 (-37.9906, -17.3066) -> (-39.8803, -17.3066)
  line L585 (-39.8803, -17.3066) -> (-39.8803, -16.3349)
  line L586 (-39.8803, -16.3349) -> (-36.386, -16.3349)
  line L587 (-36.386, -16.3349) -> (-36.386, -17.1728)
  line L588 (-36.386, -17.1728) -> (-38.3694, -19.495)
  line L589 (-38.3694, -19.495) -> (-36.3459, -19.495)
  line L590 (-36.3459, -19.495) -> (-36.3459, -20.4844)
  line L591 (-37.4245, -15.7466) -> (-38.7527, -15.7466)
  line L592 (-38.7527, -15.7466) -> (-38.7527, -14.7393)
  line L593 (-38.7527, -14.7393) -> (-37.4245, -14.7393)
  line L594 (-37.4245, -14.7393) -> (-37.4245, -15.7466)
  line L595 (-34.3402, -20.4844) -> (-35.6461, -20.4844)
  line L596 (-35.6461, -20.4844) -> (-35.6461, -19.0314)
  line L597 (-35.6461, -19.0314) -> (-34.3402, -19.0314)
  line L598 (-34.3402, -19.0314) -> (-34.3402, -20.4844)
  spline S441 degree 2 poles (-26.117, -17.7389) (-26.117, -18.51) (-26.79, -19.7223) (-27.3026, -20.0476) knots 0 0 0 1 2 2 2
  spline S442 degree 2 poles (-27.3026, -20.0476) (-27.7304, -20.324) (-28.7377, -20.4844) (-29.3038, -20.4844) knots 0 0 0 1 2 2 2
  line L599 (-29.3038, -20.4844) -> (-31.0242, -20.4844)
  line L600 (-31.0242, -20.4844) -> (-31.0242, -14.9844)
  line L601 (-31.0242, -14.9844) -> (-29.3216, -14.9844)
  spline S443 degree 2 poles (-29.3216, -14.9844) (-28.7422, -14.9844) (-27.7304, -15.1315) (-27.2847, -15.4168) knots 0 0 0 1 2 2 2
  spline S444 degree 2 poles (-27.2847, -15.4168) (-26.7454, -15.7644) (-26.117, -16.9411) (-26.117, -17.7389) knots 0 0 0 1 2 2 2
  spline S445 degree 2 poles (-27.5343, -17.73) (-27.5343, -17.1862) (-27.9087, -16.4107) (-28.292, -16.1923) knots 0 0 0 1 2 2 2
  spline S446 degree 2 poles (-28.292, -16.1923) (-28.5728, -16.0408) (-29.1879, -16.0096) (-29.6158, -16.0096) knots 0 0 0 1 2 2 2
  line L602 (-29.6158, -16.0096) -> (-29.6425, -16.0096)
  line L603 (-29.6425, -16.0096) -> (-29.6425, -19.4549)
  line L604 (-29.6425, -19.4549) -> (-29.6158, -19.4549)
  spline S447 degree 2 poles (-29.6158, -19.4549) (-29.1522, -19.4549) (-28.5149, -19.4237) (-28.2252, -19.2409) knots 0 0 0 1 2 2 2
  spline S448 degree 2 poles (-28.2252, -19.2409) (-27.8864, -19.027) (-27.5343, -18.2737) (-27.5343, -17.73) knots 0 0 0 1 2 2 2
  spline S449 degree 2 poles (-23.0862, -20.0432) (-23.2199, -20.1546) (-23.4294, -20.3329) (-23.6077, -20.422) knots 0 0 0 1 2 2 2
  spline S450 degree 2 poles (-23.6077, -20.422) (-23.7815, -20.5067) (-24.1113, -20.5959) (-24.4055, -20.5959) knots 0 0 0 1 2 2 2
  spline S451 degree 2 poles (-24.4055, -20.5959) (-24.9581, -20.5959) (-25.6846, -19.856) (-25.6846, -19.2944) knots 0 0 0 1 2 2 2
  spline S452 degree 2 poles (-25.6846, -19.2944) (-25.6846, -18.8353) (-25.3147, -18.2648) (-24.9671, -18.0999) knots 0 0 0 1 2 2 2
  spline S453 degree 2 poles (-24.9671, -18.0999) (-24.615, -17.9305) (-23.6389, -17.7968) (-23.0773, -17.7612) knots 0 0 0 1 2 2 2
  line L605 (-23.0773, -17.7612) -> (-23.0773, -17.7389)
  spline S454 degree 2 poles (-23.0773, -17.7389) (-23.0773, -17.3957) (-23.5854, -17.1327) (-24.0935, -17.1327) knots 0 0 0 1 2 2 2
  spline S455 degree 2 poles (-24.0935, -17.1327) (-24.3208, -17.1327) (-24.9359, -17.2976) (-25.2256, -17.4269) knots 0 0 0 1 2 2 2
  line L606 (-25.2256, -17.4269) -> (-25.337, -17.4269)
  line L607 (-25.337, -17.4269) -> (-25.337, -16.4241)
  spline S456 degree 2 poles (-25.337, -16.4241) (-25.1453, -16.3706) (-24.2896, -16.219) (-23.8528, -16.219) knots 0 0 0 1 2 2 2
  spline S457 degree 2 poles (-23.8528, -16.219) (-22.7831, -16.219) (-21.8026, -16.9322) (-21.8026, -17.6631) knots 0 0 0 1 2 2 2
  line L608 (-21.8026, -17.6631) -> (-21.8026, -20.4844)
  line L609 (-21.8026, -20.4844) -> (-23.0862, -20.4844)
  line L610 (-23.0862, -20.4844) -> (-23.0862, -20.0432)
  line L611 (-23.0862, -19.4014) -> (-23.0862, -18.5412)
  spline S458 degree 2 poles (-23.0862, -18.5412) (-23.416, -18.5724) (-23.8216, -18.6214) (-24.0177, -18.6927) knots 0 0 0 1 2 2 2
  spline S459 degree 2 poles (-24.0177, -18.6927) (-24.1915, -18.7506) (-24.3787, -18.9913) (-24.3787, -19.1874) knots 0 0 0 1 2 2 2
  spline S460 degree 2 poles (-24.3787, -19.1874) (-24.3787, -19.4771) (-24.0623, -19.6955) (-23.7547, -19.6955) knots 0 0 0 1 2 2 2
  spline S461 degree 2 poles (-23.7547, -19.6955) (-23.5854, -19.6955) (-23.2288, -19.5395) (-23.0862, -19.4014) knots 0 0 0 1 2 2 2
  line L612 (-18.0586, -17.5606) -> (-18.1656, -17.5606)
  spline S462 degree 2 poles (-18.1656, -17.5606) (-18.2414, -17.5339) (-18.5222, -17.5071) (-18.6915, -17.5071) knots 0 0 0 1 2 2 2
  spline S463 degree 2 poles (-18.6915, -17.5071) (-18.8921, -17.5071) (-19.3423, -17.6275) (-19.5517, -17.7077) knots 0 0 0 1 2 2 2
  line L613 (-19.5517, -17.7077) -> (-19.5517, -20.4844)
  line L614 (-19.5517, -20.4844) -> (-20.8443, -20.4844)
  line L615 (-20.8443, -20.4844) -> (-20.8443, -16.3349)
  line L616 (-20.8443, -16.3349) -> (-19.5517, -16.3349)
  line L617 (-19.5517, -16.3349) -> (-19.5517, -16.9322)
  spline S464 degree 2 poles (-19.5517, -16.9322) (-19.4626, -16.8519) (-19.1506, -16.6023) (-19.0214, -16.5266) knots 0 0 0 1 2 2 2
  spline S465 degree 2 poles (-19.0214, -16.5266) (-18.8787, -16.4419) (-18.5043, -16.3216) (-18.3394, -16.3216) knots 0 0 0 1 2 2 2
  spline S466 degree 2 poles (-18.3394, -16.3216) (-18.277, -16.3216) (-18.121, -16.3305) (-18.0586, -16.3349) knots 0 0 0 1 2 2 2
  line L618 (-18.0586, -16.3349) -> (-18.0586, -17.5606)
  line L619 (-16.2714, -20.4844) -> (-17.5639, -20.4844)
  line L620 (-17.5639, -20.4844) -> (-17.5639, -16.3349)
  line L621 (-17.5639, -16.3349) -> (-16.2714, -16.3349)
  line L622 (-16.2714, -16.3349) -> (-16.2714, -20.4844)
  line L623 (-16.2312, -15.7421) -> (-17.5996, -15.7421)
  line L624 (-17.5996, -15.7421) -> (-17.5996, -14.7348)
  line L625 (-17.5996, -14.7348) -> (-16.2312, -14.7348)
  line L626 (-16.2312, -14.7348) -> (-16.2312, -15.7421)
  line L627 (-11.431, -20.4844) -> (-12.7235, -20.4844)
  line L628 (-12.7235, -20.4844) -> (-12.7235, -20.0254)
  spline S467 degree 2 poles (-12.7235, -20.0254) (-13.0578, -20.3062) (-13.6194, -20.6003) (-14.0072, -20.6003) knots 0 0 0 1 2 2 2
  spline S468 degree 2 poles (-14.0072, -20.6003) (-14.6222, -20.6003) (-15.3131, -19.8203) (-15.3131, -19.0359) knots 0 0 0 1 2 2 2
  line L629 (-15.3131, -19.0359) -> (-15.3131, -16.3349)
  line L630 (-15.3131, -16.3349) -> (-14.0116, -16.3349)
  line L631 (-14.0116, -16.3349) -> (-14.0116, -18.3941)
  spline S469 degree 2 poles (-14.0116, -18.3941) (-14.0116, -18.715) (-13.9804, -19.125) (-13.918, -19.2632) knots 0 0 0 1 2 2 2
  spline S470 degree 2 poles (-13.918, -19.2632) (-13.8556, -19.3925) (-13.6105, -19.5262) (-13.3876, -19.5262) knots 0 0 0 1 2 2 2
  spline S471 degree 2 poles (-13.3876, -19.5262) (-13.2539, -19.5262) (-12.8795, -19.3925) (-12.7235, -19.2766) knots 0 0 0 1 2 2 2
  line L632 (-12.7235, -19.2766) -> (-12.7235, -16.3349)
  line L633 (-12.7235, -16.3349) -> (-11.431, -16.3349)
  line L634 (-11.431, -16.3349) -> (-11.431, -20.4844)
  spline S472 degree 2 poles (-9.1802, -20.5959) (-9.6348, -20.5959) (-10.4504, -20.3953) (-10.7179, -20.2616) knots 0 0 0 1 2 2 2
  line L635 (-10.7179, -20.2616) -> (-10.7179, -19.1696)
  line L636 (-10.7179, -19.1696) -> (-10.6109, -19.1696)
  spline S473 degree 2 poles (-10.6109, -19.1696) (-10.5173, -19.2409) (-10.2811, -19.4103) (-10.0716, -19.5039) knots 0 0 0 1 2 2 2
  spline S474 degree 2 poles (-10.0716, -19.5039) (-9.8889, -19.5886) (-9.4387, -19.7089) (-9.1713, -19.7089) knots 0 0 0 1 2 2 2
  spline S475 degree 2 poles (-9.1713, -19.7089) (-8.8994, -19.7089) (-8.4804, -19.5395) (-8.4804, -19.3568) knots 0 0 0 1 2 2 2
  spline S476 degree 2 poles (-8.4804, -19.3568) (-8.4804, -19.2142) (-8.6721, -19.0626) (-8.9484, -19.0002) knots 0 0 0 1 2 2 2
  spline S477 degree 2 poles (-8.9484, -19.0002) (-9.0955, -18.9601) (-9.5457, -18.8754) (-9.7195, -18.822) knots 0 0 0 1 2 2 2
  spline S478 degree 2 poles (-9.7195, -18.822) (-10.2098, -18.6704) (-10.7, -18.0776) (-10.7, -17.5918) knots 0 0 0 1 2 2 2
  spline S479 degree 2 poles (-10.7, -17.5918) (-10.7, -17.3155) (-10.446, -16.8252) (-10.1964, -16.6335) knots 0 0 0 1 2 2 2
  spline S480 degree 2 poles (-10.1964, -16.6335) (-9.9513, -16.4463) (-9.2248, -16.2235) (-8.7657, -16.2235) knots 0 0 0 1 2 2 2
  spline S481 degree 2 poles (-8.7657, -16.2235) (-8.3289, -16.2235) (-7.5979, -16.3973) (-7.3483, -16.5177) knots 0 0 0 1 2 2 2
  line L637 (-7.3483, -16.5177) -> (-7.3483, -17.5695)
  line L638 (-7.3483, -17.5695) -> (-7.4508, -17.5695)
  spline S482 degree 2 poles (-7.4508, -17.5695) (-7.5177, -17.516) (-7.8074, -17.3422) (-7.9411, -17.2798) knots 0 0 0 1 2 2 2
  spline S483 degree 2 poles (-7.9411, -17.2798) (-8.106, -17.2085) (-8.5072, -17.1104) (-8.7167, -17.1104) knots 0 0 0 1 2 2 2
  spline S484 degree 2 poles (-8.7167, -17.1104) (-8.9974, -17.1104) (-9.3852, -17.3021) (-9.3852, -17.4581) knots 0 0 0 1 2 2 2
  spline S485 degree 2 poles (-9.3852, -17.4581) (-9.3852, -17.6007) (-9.1936, -17.7612) (-8.8726, -17.8414) knots 0 0 0 1 2 2 2
  spline S486 degree 2 poles (-8.8726, -17.8414) (-8.7077, -17.8815) (-8.2754, -17.9573) (-8.0748, -18.0241) knots 0 0 0 1 2 2 2
  spline S487 degree 2 poles (-8.0748, -18.0241) (-7.6291, -18.1668) (-7.1656, -18.7239) (-7.1656, -19.1874) knots 0 0 0 1 2 2 2
  spline S488 degree 2 poles (-7.1656, -19.1874) (-7.1656, -19.4771) (-7.4375, -20.0075) (-7.6915, -20.1858) knots 0 0 0 1 2 2 2
  spline S489 degree 2 poles (-7.6915, -20.1858) (-7.9545, -20.3819) (-8.6765, -20.5959) (-9.1802, -20.5959) knots 0 0 0 1 2 2 2
  line L639 (-3.2434, -20.4844) -> (-6.867, -20.4844)
  line L640 (-6.867, -20.4844) -> (-6.867, -19.6331)
  line L641 (-6.867, -19.6331) -> (-4.888, -17.3066)
  line L642 (-4.888, -17.3066) -> (-6.7778, -17.3066)
  line L643 (-6.7778, -17.3066) -> (-6.7778, -16.3349)
  line L644 (-6.7778, -16.3349) -> (-3.2835, -16.3349)
  line L645 (-3.2835, -16.3349) -> (-3.2835, -17.1728)
  line L646 (-3.2835, -17.1728) -> (-5.2669, -19.495)
  line L647 (-5.2669, -19.495) -> (-3.2434, -19.495)
  line L648 (-3.2434, -19.495) -> (-3.2434, -20.4844)
  spline S490 degree 2 poles (-0.2884, -20.0432) (-0.4221, -20.1546) (-0.6316, -20.3329) (-0.8098, -20.422) knots 0 0 0 1 2 2 2
  spline S491 degree 2 poles (-0.8098, -20.422) (-0.9837, -20.5067) (-1.3135, -20.5959) (-1.6077, -20.5959) knots 0 0 0 1 2 2 2
  spline S492 degree 2 poles (-1.6077, -20.5959) (-2.1603, -20.5959) (-2.8868, -19.856) (-2.8868, -19.2944) knots 0 0 0 1 2 2 2
  spline S493 degree 2 poles (-2.8868, -19.2944) (-2.8868, -18.8353) (-2.5169, -18.2648) (-2.1692, -18.0999) knots 0 0 0 1 2 2 2
  spline S494 degree 2 poles (-2.1692, -18.0999) (-1.8171, -17.9305) (-0.841, -17.7968) (-0.2795, -17.7612) knots 0 0 0 1 2 2 2
  line L649 (-0.2795, -17.7612) -> (-0.2795, -17.7389)
  spline S495 degree 2 poles (-0.2795, -17.7389) (-0.2795, -17.3957) (-0.7876, -17.1327) (-1.2957, -17.1327) knots 0 0 0 1 2 2 2
  spline S496 degree 2 poles (-1.2957, -17.1327) (-1.523, -17.1327) (-2.138, -17.2976) (-2.4278, -17.4269) knots 0 0 0 1 2 2 2
  line L650 (-2.4278, -17.4269) -> (-2.5392, -17.4269)
  line L651 (-2.5392, -17.4269) -> (-2.5392, -16.4241)
  spline S497 degree 2 poles (-2.5392, -16.4241) (-2.3475, -16.3706) (-1.4918, -16.219) (-1.055, -16.219) knots 0 0 0 1 2 2 2
  spline S498 degree 2 poles (-1.055, -16.219) (0.0147, -16.219) (0.9953, -16.9322) (0.9953, -17.6631) knots 0 0 0 1 2 2 2
  line L652 (0.9953, -17.6631) -> (0.9953, -20.4844)
  line L653 (0.9953, -20.4844) -> (-0.2884, -20.4844)
  line L654 (-0.2884, -20.4844) -> (-0.2884, -20.0432)
  line L655 (-0.2884, -19.4014) -> (-0.2884, -18.5412)
  spline S499 degree 2 poles (-0.2884, -18.5412) (-0.6182, -18.5724) (-1.0238, -18.6214) (-1.2199, -18.6927) knots 0 0 0 1 2 2 2
  spline S500 degree 2 poles (-1.2199, -18.6927) (-1.3937, -18.7506) (-1.5809, -18.9913) (-1.5809, -19.1874) knots 0 0 0 1 2 2 2
  spline S501 degree 2 poles (-1.5809, -19.1874) (-1.5809, -19.4771) (-1.2645, -19.6955) (-0.9569, -19.6955) knots 0 0 0 1 2 2 2
  spline S502 degree 2 poles (-0.9569, -19.6955) (-0.7876, -19.6955) (-0.431, -19.5395) (-0.2884, -19.4014) knots 0 0 0 1 2 2 2
  line L656 (9.8603, -20.4844) -> (8.4876, -20.4844)
  line L657 (8.4876, -20.4844) -> (8.4876, -16.8386)
  line L658 (8.4876, -16.8386) -> (7.4892, -19.1919)
  line L659 (7.4892, -19.1919) -> (6.5443, -19.1919)
  line L660 (6.5443, -19.1919) -> (5.5459, -16.8386)
  line L661 (5.5459, -16.8386) -> (5.5459, -20.4844)
  line L662 (5.5459, -20.4844) -> (4.2445, -20.4844)
  line L663 (4.2445, -20.4844) -> (4.2445, -14.9844)
  line L664 (4.2445, -14.9844) -> (5.8356, -14.9844)